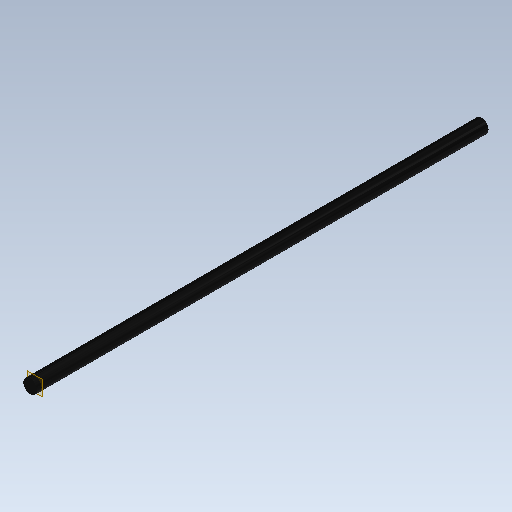
# Autodesk Inventor part: ADSK-MH-10023
Saved by Autodesk Inventor 2020.2 (Build 242310000, 310)
## iProperties
Created: 2008-03-10
Part Number: ADSK-MH-10023
Document SubType Name: Modeling
Designer: R.O'mahony
Density: 7.86 g/cm^3
Mass: 17.5487 g
Surface Area: 58.6103 cm^2
Volume: 17.5487 cm^3
Material: Steel, Mild
Appearance: Glossy - Black
Description: Roller Component
Engineer: Demir Ali
Checked By: Demir Ali
Company: Autodesk Ltd
Author: R.O'mahony
Keywords: Roller Conveyor
Revision Number: A
Autodesk Inventor part; units mm, degrees
ref_plane "YZ Plane" through (0, 0, 0) normal (1, 0, 0) x (0, 1, 0)
ref_plane "XZ Plane" through (0, 0, 0) normal (0, 1, 0) x (-1, 0, 0)
ref_plane "XY Plane" through (0, 0, 0) normal (0, 0, 1) x (1, 0, 0)
sketch "Sketch1" plane through (0, 0, 0) normal (0, 0, 1) x (1, 0, 0)
  circle A0 centre (0, 0) radius 6.25
  dimension "d0" = 12.5
  constraints: 1 centre point, 1 coincident
  measures "d0" diameter of A0
extrude "Extrusion1" add sketch "Sketch1" along normal mid plane 408
ref_plane "Work Plane1" through (0, 0, 200) normal (0, 0, 1) x (1, 0, 0)
equation "\"d1\" = Roller_width"
equation "\"Roller_width\" = 408"
body "Solid1"
